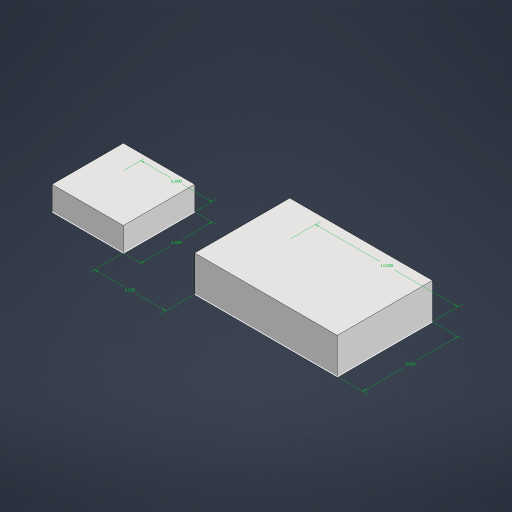
# Autodesk Inventor part: Part4
Saved by Autodesk Inventor 2023.1 (Build 271208000, 208)
## iProperties
RuleStatus: InUse
Created: 2022-11-09
Part Number: Part4
Material: Generic
Document SubType Name: Modeling
Designer: awelt
Mass: 5899.34 g
Surface Area: 2787.09 cm^2
Volume: 5899.34 cm^3
Density: 1 g/cm^3
Appearance: Default
BeforeDocSave0: file://C:\Users\awelt\Documents\Inventor\iLogic_Rules\BoundingStore
DocClose0: file://C:\Users\awelt\Documents\Inventor\iLogic_Rules\BoundingStore
BoundingBL1: 3
BoundingBL2: 8
BoundingBL3: 24
BoundingCF: 0.333
Author: awelt
Autodesk Inventor part; units mm, degrees
ref_plane "YZ Plane" through (0, 0, 0) normal (1, 0, 0) x (0, 1, 0)
ref_plane "XZ Plane" through (0, 0, 0) normal (0, 1, 0) x (-1, 0, 0)
ref_plane "XY Plane" through (0, 0, 0) normal (0, 0, 1) x (1, 0, 0)
sketch "Sketch2" plane through (0, 0, 0) normal (0, 1, 0) x (-1, 0, 0)
  line L0 (0, 0) -> (-152.4, 0)
  line L1 (-152.4, 0) -> (-152.4, -152.4)
  line L2 (-152.4, -152.4) -> (0, -152.4)
  line L3 (0, -152.4) -> (0, 0)
  line L4 (-304.8, 0) -> (-609.6, 0)
  line L5 (-609.6, 0) -> (-609.6, -203.2)
  line L6 (-609.6, -203.2) -> (-304.8, -203.2)
  line L7 (-304.8, -203.2) -> (-304.8, 0)
  dimension "d3" = 152.4
  dimension "d4" = 152.4
  dimension "d7" = 304.8
  dimension "d8" = 203.2
  dimension "d9" = 152.4
  constraints: 16 end point, 4 parallel, 2 horizontal, 2 perpendicular, 1 collinear
  measures "d3" distance of L2.end L1.end
  measures "d4" distance of L1.end L0.end
  measures "d7" distance of L6.end L5.end
  measures "d8" distance of L5.end L4.end
  measures "d9" distance of L4.start L0.end
extrude "Extrusion1" add sketch "Sketch2" along normal blind 50.8 contours L3 L2 L1 L0
extrude "Extrusion2" add sketch "Sketch2" along normal blind 76.2 separate body contours L7 L6 L5 L4
body "Solid1"
body "Solid2"
